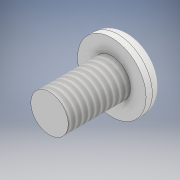
# Autodesk Inventor part: 4mmScrew
Saved by Autodesk Inventor 2017 (Build 210142000, 142)
## iProperties
Created: 2019-03-18
Part Number: 4mmScrew
Material: Generic
Document SubType Name: Modeling
Designer: cresswnd
Density: 1 g/cm^3
Appearance: White
Author: cresswnd
Autodesk Inventor part; units mm, degrees
ref_plane "YZ Plane" through (0, 0, 0) normal (1, 0, 0) x (0, 1, 0)
ref_plane "XZ Plane" through (0, 0, 0) normal (0, 1, 0) x (-1, 0, 0)
ref_plane "XY Plane" through (0, 0, 0) normal (0, 0, 1) x (1, 0, 0)
sketch "Sketch1" plane through (0, 0, 0) normal (0, 1, 0) x (-1, 0, 0)
  circle A0 centre (0, 0) radius 1.5
  dimension "d0" = 3
  constraints: 1 centre point, 1 coincident
  measures "d0" diameter of A0
extrude "Extrusion1" add sketch "Sketch1" along normal blind 5
sketch "Sketch2" plane through (0, 5, 0) normal (0, 1, 0) x (1, 0, 0)
  circle A0 centre (0, 0) radius 1.25 construction
  line L0 (-1.25, 0) -> (-0.625, 1.0825)
  line L1 (-0.625, 1.0825) -> (0.625, 1.0825)
  line L2 (0.625, 1.0825) -> (1.25, 0)
  line L3 (1.25, 0) -> (0.625, -1.0825)
  line L4 (0.625, -1.0825) -> (-0.625, -1.0825)
  line L5 (-0.625, -1.0825) -> (-1.25, 0)
  circle A1 centre (0, 0) radius 2.75
  dimension "d3" = 2.5
  dimension "d4" = 5.5
  constraints: 12 end point, 3 coincident, 1 centre point, 1 horizontal alignment, 15 other
  measures "d4" diameter of A1
extrude "Extrusion2" add sketch "Sketch2" along normal blind 1.5
fillet "Fillet1" radius 1 1 edges at (-2.75, 6.5, 0)
thread "Thread1" size "M3x0.5" class "6g" standard "ANSI Metric M Profile" full length
body "Solid1"
